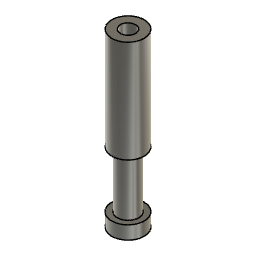
AirTankPlug v1 (Autodesk Fusion 360 design; units mm, degrees)
Autodesk Fusion 360 part; units mm, degrees
sketch "Sketch1" plane through (0, 0, 0) normal (0, 0, 1) x (1, 0, 0)
  circle A0 centre (0, 0) radius 3.175
  dimension "d1" = 6.35
  constraint coincident A0.centre origin
  measures "d1" diameter of A0
extrude "Extrude1" add sketch "Sketch1" along normal blind 2.6
sketch "Sketch2" plane through (0, 0, 2.6) normal (0, 0, 1) x (-1, 0, 0)
  circle A0 centre (0, 0) radius 3.175
  circle A1 centre (0, 0) radius 2.0955
  dimension "d4" = 4.191
  constraint coincident A0.centre A1.centre
  measures "d4" diameter of A1
extrude "Extrude2" add sketch "Sketch2" along normal blind 11 contours A1
sketch "Sketch3" plane through (0, 0, 13.6) normal (0, 0, 1) x (-1, 0, 0)
  circle A0 centre (0, 0) radius 2.0955
  circle A1 centre (0, 0) radius 3.175
  dimension "d7" = 6.35
  constraint coincident A0.centre A1.centre
  measures "d7" diameter of A1
extrude "Extrude3" add sketch "Sketch3" along normal blind 20 contours A0 | A1
sketch "Sketch4" plane through (0, 0, 33.6) normal (0, 0, 1) x (-1, 0, 0)
  circle A0 centre (0, 0) radius 3.175
  circle A1 centre (0, 0) radius 1.5
  dimension "d10" = 3
  constraint coincident A0.centre A1.centre
  measures "d10" diameter of A1
extrude "Extrude4" cut sketch "Sketch4" against normal blind 15 contours A1
